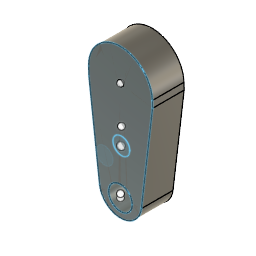
LEG 1 (Autodesk Fusion 360 design; units mm, degrees)
part number: 2026-03-06-00-13-43-154
Autodesk Fusion 360 part; units mm, degrees
sketch "Sketch1" plane through (0, 0, 0) normal (0, 1, 0) x (1, 0, 0)
  line L0 (36.6393, -44.8476) -> (36.8758, -36.9029)
  line L1 (-38.7425, -32.3133) -> (-39.0485, -42.5947)
  arc A0 (-39.0485, -42.5947) -> (36.6393, -44.8476) centre (-1.2046, -43.7212) ccw
  circle A1 centre (-1.2046, -43.7212) radius 3.5
  circle A2 centre (-1.2046, 74.3196) radius 14
  line L2 (36.8758, -36.9029) -> (23.6155, 73.0203)
  line L3 (-38.7425, -32.3133) -> (-26.0243, 73.0229)
  arc A3 (23.6155, 73.0203) -> (13.7954, 90.0262) centre (-1.2046, 70.0262) ccw
  arc A4 (13.7954, 90.0262) -> (-26.0243, 73.0229) centre (-1.2046, 70.0262) ccw
  dimension "d11" = 28
  dimension "d12" = 25
  dimension "d13" = 25
  dimension "d14" = 105.3362
  dimension "d29" = 7
  constraint parallel L0 L1
  constraint tangent L1 A0
  constraint tangent L0 A0
  constraint concentric A0 A1
  constraint tangent L2 A3
  constraint tangent L3 A4
  constraint tangent A3 A4
  measures "d11" diameter of A2
  measures "d12" radius of A3
  measures "d13" radius of A4
  measures "d14" vertical distance of L1.start L3.end
  measures "d29" diameter of A1
sketch "Sketch2" plane through (0, 0, 0) normal (0, 1, 0) x (1, 0, 0)
  arc A0 (13.7954, 90.0262) -> (-26.0243, 73.0229) centre (-1.2046, 70.0262) ccw
  line L0 (-38.7425, -32.3133) -> (-39.0485, -42.5947)
  arc A1 (23.6155, 73.0203) -> (13.7954, 90.0262) centre (-1.2046, 70.0262) ccw
  circle A2 centre (-1.2046, 74.3196) radius 14
  line L1 (36.8758, -36.9029) -> (23.6155, 73.0203)
  line L2 (-38.7425, -32.3133) -> (-26.0243, 73.0229)
  arc A3 (-39.0485, -42.5947) -> (36.6393, -44.8476) centre (-1.2046, -43.7212) ccw
  line L3 (36.6393, -44.8476) -> (36.8758, -36.9029)
  dimension "d17" = 28
  dimension "d18" = 25
  dimension "d19" = 25
  dimension "d20" = 105.3362
  constraint parallel L0 L3
  constraint tangent L0 A3
  constraint tangent A3 L3
  constraint tangent A1 L1
  constraint tangent A0 L2
  constraint tangent A0 A1
  measures "d17" diameter of A2
  measures "d18" radius of A1
  measures "d19" radius of A0
  measures "d20" vertical distance of L0.start A0.end
sketch "Sketch3" plane through (0, 0, 0) normal (0, 1, 0) x (1, 0, 0)
  circle A0 centre (0, 20) radius 10
  dimension "d21" = 20
  measures "d21" diameter of A0
sketch "Sketch4" plane through (0, -20, 0) normal (0, -1, 0) x (1, 0, 0)
  circle A0 centre (0, -20) radius 10
extrude "Extrude5" add sketch "Sketch1" along normal blind 37.67
equation "d11 = 0.056 m / 2"
